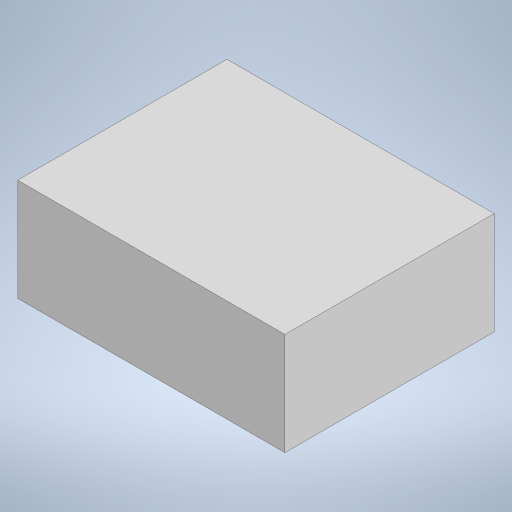
# Autodesk Inventor part: CH-1-01-motorController
Saved by Autodesk Inventor 2023 (Build 270158000, 158)
## iProperties
Created: 2022-11-15
Part Number: CH-1-01-motorController
Material: Generic
Document SubType Name: Modeling
Designer: megan
Density: 1 g/cm^3
Appearance: Default
Author: megan
Autodesk Inventor part; units mm, degrees
ref_plane "YZ Plane" through (0, 0, 0) normal (1, 0, 0) x (0, 1, 0)
ref_plane "XZ Plane" through (0, 0, 0) normal (0, 1, 0) x (-1, 0, 0)
ref_plane "XY Plane" through (0, 0, 0) normal (0, 0, 1) x (1, 0, 0)
sketch "Sketch1" plane through (0, 0, 0) normal (0, 1, 0) x (-1, 0, 0)
  line L0 (30, 23.5) -> (-30, 23.5)
  line L1 (-30, 23.5) -> (-30, -23.5)
  line L2 (-30, -23.5) -> (30, -23.5)
  line L3 (30, -23.5) -> (30, 23.5)
  line L4 (30, 23.5) -> (-30, -23.5) construction
  line L5 (-30, 23.5) -> (30, -23.5) construction
  point P0 (0, 0)
  dimension "d0" = 47
  dimension "d1" = 60
  constraints: 12 end point, 2 midpoint, 2 parallel, 1 horizontal, 1 perpendicular
  measures "d0" distance between parallel lines of L2 L0
  measures "d1" distance between parallel lines of L1 L3
extrude "Extrusion1" add sketch "Sketch1" along normal blind 23
body "Solid1"
